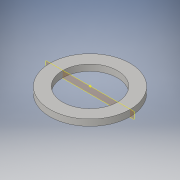
# Autodesk Inventor part: vexCam5
Saved by Autodesk Inventor 2016 SP1 (Build 200210100, 210)
## iProperties
Created: 2015-07-25
Part Number: vexCam5
Material: Generic
Document SubType Name: Modeling
Designer: steele
Density: 1 g/cm^3
Appearance: Default
Author: steele
Autodesk Inventor part; units mm, degrees
ref_plane "YZ Plane" through (0, 0, 0) normal (1, 0, 0) x (0, 1, 0)
ref_plane "XZ Plane" through (0, 0, 0) normal (0, 1, 0) x (-1, 0, 0)
sketch "Sketch1" plane through (0, 0, 0) normal (0, 1, 0) x (-1, 0, 0)
  circle A0 centre (0, 0) radius 55.0333
  circle A1 centre (0, 0) radius 80.4333
  dimension "insideCamDiam" = 110.0667
  dimension "outsideCamDiam" = 160.8667
  constraints: 2 centre point, 1 coincident
  measures "insideCamDiam" diameter of A0
  measures "outsideCamDiam" diameter of A1
extrude "Extrusion1" add sketch "Sketch1" against normal blind 12.7
equation "\"frisbeeOuterDiamter\" = 105.83333"
equation "\"frisbeeHopperOutsideDiam\" = 97.36667"
equation "\"one_third_of_circle\" = 120deg"
equation "\"camTrackDiam\" = 6.35"
equation "\"camRadius\" = 74.08333"
body "Solid1"
